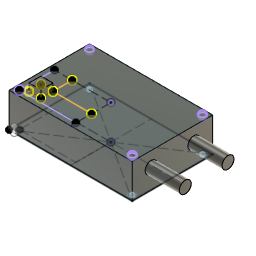
Redesign of Circuit Housing for Cthulhu v8 (Autodesk Fusion 360 archive; units mm, degrees)
design "Housing for Cthulu Lamp"
Autodesk Fusion 360 part; units mm, degrees
sketch "Board size" plane through (0, 0, 0) normal (0, 0, 1) x (1, 0, 0)
  line L0 (36, 23.5) -> (-36, 23.5)
  line L1 (-36, 23.5) -> (-36, -23.5)
  line L2 (-36, -23.5) -> (36, -23.5)
  line L3 (36, -23.5) -> (36, 23.5)
  line L4 (36, 23.5) -> (-36, -23.5) construction
  line L5 (-36, 23.5) -> (36, -23.5) construction
  dimension "d1" = 72
  dimension "d2" = 47
  constraint horizontal L0
  constraint perpendicular L0 L1
  constraint parallel L0 L2
  constraint parallel L1 L3
  constraint coincident L4 origin
  constraint coincident L5 origin
  measures "d1" distance of L1.end L2.end
  measures "d2" distance of L0.end L1.end
sketch "Pot side" plane through (36, 0, 0) normal (1, 0, 0) x (0, 1, 0)
  line L0 (-23.5, 0) -> (23.5, 0)
  line L1 (23.5, 0) -> (23.5, 22)
  line L2 (23.5, 22) -> (-23.5, 22)
  line L3 (-23.5, 22) -> (-23.5, 0)
  circle A0 centre (-12.5, 11.5) radius 3.5
  line L4 (0, 0) -> (0, 22) construction
  circle A1 centre (12.5, 11.5) radius 3.5
  line L5 (0, 0) -> (-12.5, 0)
  line L6 (-12.5, 0) -> (-12.5, 11.5) construction
  line L7 (-12.5, 11.5) -> (0, 11.5) construction
  line L8 (0, 11.5) -> (0, 0)
  dimension "d7" = 7
  dimension "d20" = 12.5
  dimension "d21" = 11.5
  constraint coincident L4.start L5.start
  constraint midpoint L2 L4.end
  constraint symmetric A0 L4 A1
  constraint horizontal L5
  constraint vertical L6
  constraint horizontal L7
  constraint vertical L8
  constraint coincident A0.centre L7
  constraint coincident A0.centre L6
  measures "d7" diameter of A0
  measures "d20" distance of L4.start L5.end
  measures "d21" distance of L4.start L7.end
sketch "Sketch3" plane through (0, 0, 0) normal (0, 0, -1) x (1, 0, 0)
  line L0 (36, -23.5) -> (36, 23.5)
  line L1 (36, 23.5) -> (-36, 23.5)
  line L2 (-36, 23.5) -> (-36, -23.5)
  line L3 (-36, -23.5) -> (36, -23.5)
  line L4 (-36, 23.5) -> (-33, 23.5)
  line L5 (-36, 20.5) -> (-36, 23.5)
  circle A0 centre (-33, 20.5) radius 1.7
  line L6 (-36, 0) -> (36, 0) construction
  line L7 (0, 23.5) -> (0, -23.5) construction
  circle A1 centre (33, 20.5) radius 1.7
  circle A2 centre (33, -20.5) radius 1.7
  circle A3 centre (-33, -20.5) radius 1.7
  line L8 (0, 0) -> (-33, 0) construction
  line L9 (-33, 0) -> (-33, 20.5) construction
  line L10 (-33, 20.5) -> (0, 20.5) construction
  line L11 (0, 20.5) -> (0, 0) construction
  dimension "d10" = 3.4
  dimension "d23" = 33
  dimension "d24" = 20.5
  constraint coincident L1.end L2.start
  constraint midpoint L2 L6.start
  constraint midpoint L0 L6.end
  constraint midpoint L1 L7.start
  constraint midpoint L3 L7.end
  constraint symmetric L6 A1 A2
  constraint horizontal L8
  constraint vertical L9
  constraint horizontal L10
  constraint vertical L11
  constraint coincident L8.start L11.end
  constraint coincident A0.centre L10
  constraint coincident A0.centre L9
  measures "d10" diameter of A0
  measures "d23" distance of L8.start L8.end
  measures "d24" distance of L8.start L10.end
extrude "Extrude1" add sketch "Board size" along normal blind 20 makes body 1 in component "Box"
extrude "Extrude9" add sketch "Pot side" along normal blind 20 contours A0 | A1 bodies 1 in component "Box"
extrude "Extrude1'" add sketch "Board size" along normal blind 20 separate body makes body 2 in component "Lid"
shell "Shell1" thickness 2.5 removed faces 4 at (-12, -23.5, 6.6667) at (-36, 7.8333, 6.6667) at (12, 23.5, 6.6667) at (-12, 7.8333, 0) on bodies 2 in component "Lid"
extrude "Extrude2" cut sketch "Pot side" against normal blind 2.5 contours A0 | A1 bodies 2 in component "Lid"
sketch "Sketch1" plane through (0, -23.5, 0) normal (0, -1, 0) x (1, 0, 0) in component "Box"
  line L0 (-36, 0) -> (36, 0)
  line L1 (36, 0) -> (36, 20)
  line L2 (36, 20) -> (-36, 20)
  line L3 (-36, 20) -> (-36, 0)
  line L4 (36, 0) -> (36, 2.5)
  line L5 (36, 2.5) -> (34.5, 1)
  line L6 (34.5, 1) -> (34.5, 22.0494)
  line L7 (36, 22.0494) -> (34.5, 22.0494)
  line L8 (34.5, 1.5) -> (35, 1.5)
  dimension "d76" = 45
  constraint coincident L0.end L1.start
  constraint coincident L1 L4.end
  constraint perpendicular L0 L4
  constraint parallel L4 L6
  constraint coincident L1 L7.start
  constraint perpendicular L6 L7
  constraint coincident L6 L8.start
  constraint coincident L5 L8.end
  constraint perpendicular L6 L8
  measures "d76" angle of L4 L5
sketch "Sketch8" plane through (0, 0, 20) normal (0, 0, 1) x (-1, 0, 0)
  line L0 (-36, 23.5) -> (-36, -23.5)
  line L1 (-36, -23.5) -> (36, -23.5)
  line L2 (36, -23.5) -> (36, 23.5)
  line L3 (36, 23.5) -> (-36, 23.5)
  line L4 (22.6, 18.3) -> (22.6, 11.3)
  line L5 (29.6, 18.3) -> (22.6, 18.3)
  line L6 (29.6, 11.3) -> (29.6, 18.3)
  line L7 (22.6, 11.3) -> (29.6, 11.3)
  line L8 (22.6, 11.3) -> (0, 11.3)
  line L9 (22.6, 0) -> (22.6, 11.3)
  circle A0 centre (33, -20.5) radius 1.7
  circle A1 centre (-33, -20.5) radius 1.7
  circle A2 centre (33, 20.5) radius 1.7
  line L10 (33, 0) -> (33, 20.5)
  line L11 (33, 20.5) -> (0, 20.5)
  line L12 (0, 0) -> (0, 23.5) construction
  line L13 (0, 0) -> (36, 0) construction
  line L14 (0, 11.3) -> (22.6, 11.3) construction
  line L15 (22.6, 0) -> (22.6, 11.3) construction
  line L16 (33, 0) -> (33, 20.5) construction
  line L17 (0, 20.5) -> (33, 20.5) construction
  line L18 (29.6, 11.3) -> (22.6, 11.3)
  line L19 (22.6, 11.3) -> (22.6, 18.3)
  line L20 (22.6, 18.3) -> (29.6, 18.3)
  line L21 (29.6, 18.3) -> (29.6, 11.3)
  circle A3 centre (33, 20.5) radius 1.7
  circle A4 centre (-33, 20.5) radius 1.7
  point P0 (22.6, 0)
  point P1 (0, 11.3)
  point P2 (33, 20.5)
  point P3 (-33, -20.5)
  point P4 (-33, 20.5)
  dimension "d120" = 20.5
  dimension "d121" = 33
  constraint coincident L12.start L13.start
  constraint midpoint L3 L12.end
  constraint midpoint L2 L13.end
  constraint coincident P1 L8.end
  constraint coincident L4.end L7.start
  constraint coincident P0 L9.start
  constraint coincident L10.start L16.start
  constraint coincident P2 A2.centre
  constraint coincident L11.end L17.start
  constraint horizontal L18
  constraint vertical L19
  constraint horizontal L20
  constraint vertical L21
  constraint coincident L4.start L5.end
  constraint coincident L6.start L7.end
  constraint concentric A2 A3
  measures "d120" distance of L10.start P2
  measures "d121" distance of L11.end P2
extrude "Extrude10" add sketch "Sketch8" along normal blind 4.3 contours L4 L5 L6 L7 L18 L19 L20 L21 bodies 1 in component "Box"
sketch "Sketch9" plane through (0, 0, 0) normal (0, 0, -1) x (1, 0, 0)
copy_body "Body->Comp1" bodies 1 removing the originals makes body 3 in component "Board blus button and pots"
component "Box" placed x (1, 0, 0) y (0, 1, 0) z (0, 0, 1) at (0, 0, 0)
component "Lid" placed x (1, 0, 0) y (0, 1, 0) z (0, 0, 1) at (0, 0, 0)
component "Board blus button and pots" placed x (1, 0, 0) y (0, 1, 0) z (0, 0, 1) at (0, 0, 0) in component "Box"
equation "d1 = depth"
equation "d2 = width"
equation "d7 = PotHolesize"
equation "d10 = PostDiameter"
equation "d20 = PotdistanceFromcentre"
equation "d21 = PotHeightfrombottom"
equation "d23 = PostdistanceDepth"
equation "d24 = PostDistanceWidth"
equation "width = 47 mm"
equation "depth = 72 mm"
equation "PotHeightfrombottom = 11.5 mm"
equation "PotdistanceFromcentre = 12.5 mm"
equation "PotHolesize = 7 mm"
equation "PostDistanceWidth = 20.5 mm"
equation "PostdistanceDepth = 33 mm"
equation "PostDiameter = 3.4 mm"
equation "shell = 2.5 mm"
equation "gap = 0.2 mm"
equation "squarebuttonhole = 7 mm"
equation "squarebuttonholedistWidth = 22.6 mm"
equation "squarebuttonholedisDepth = 11.3 mm"
equation "height = 20 mm"
equation "d68 = height"
equation "d71 = height"
equation "d73 = shell"
equation "d74 = -shell"
equation "USBCableHole = 3.4 mm"
equation "d116 = gap"
named bodies: "THE THING INSIDE THE BOX"
